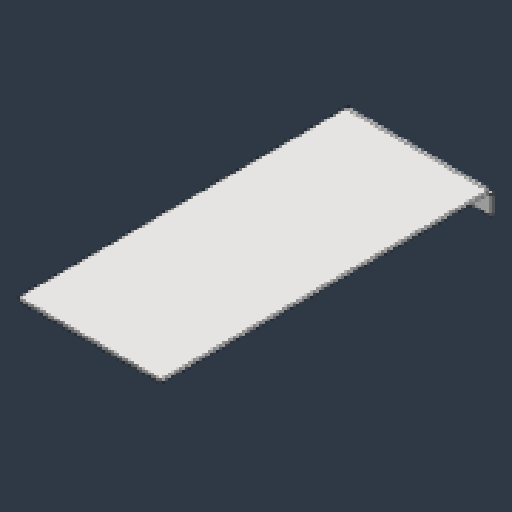
# Autodesk Inventor part: feeder_front_support
Saved by Autodesk Inventor 2024.3 (Build 283343000, 343)
## iProperties
Created: 2025-03-08
Part Number: feeder_front_support
Material: Polycarbonate, Smoke
Document SubType Name: Sheet Metal
Designer: marcu
Density: 1.2 g/cm^3
Sheet Metal Rule: Default
Appearance: Polycarbonate - Smoked
Author: marcu
Autodesk Inventor part; units mm, degrees
ref_plane "YZ Plane" through (0, 0, 0) normal (1, 0, 0) x (0, 1, 0)
ref_plane "XZ Plane" through (0, 0, 0) normal (0, 1, 0) x (-1, 0, 0)
ref_plane "XY Plane" through (0, 0, 0) normal (0, 0, 1) x (1, 0, 0)
sketch "Sketch1" plane through (0, 0, 0) normal (0, 0, 1) x (1, 0, 0)
  line L0 (76.2, -12.7) -> (-76.2, -12.7)
  line L1 (-76.2, -12.7) -> (-76.2, 12.7)
  line L2 (-76.2, 12.7) -> (76.2, 12.7)
  line L3 (76.2, 12.7) -> (76.2, -12.7)
  line L4 (76.2, -12.7) -> (-76.2, 12.7) construction
  line L5 (-76.2, -12.7) -> (76.2, 12.7) construction
  point P0 (0, 0)
  dimension "d0" = 152.4
  dimension "d1" = 25.4
  measures "d0" distance of L1.end L2.end
  measures "d1" distance of L0.end L1.end
extrude "Plate1" add sketch "Sketch1" along normal blind 3.048
sketch "Sketch2" plane through (-76.2, 9.652, 0) normal (0, 1, 0) x (-1, 0, 0)
  line L0 (-152.4, 0) -> (0, 0)
  line L1 (0, 0) -> (0, 336.55)
  line L2 (0, 336.55) -> (-152.4, 336.55)
  line L3 (-152.4, 336.55) -> (-152.4, 0)
  constraints: 6 end point, 1 horizontal, 1 perpendicular, 1 vertical
edge flange "Flange1" height 336.55 angle 90 thickness 3.048 bend radius 3.048 thickness toward (0, 1, 0) relief straight relief width 3.048 relief depth 1.524 edges at (0, 12.7, 3.048) wall of the first edge with corners at (76.2, 9.652, 0) (-76.2, 9.652, 0) (-76.2, 9.652, 336.55) (76.2, 9.652, 336.55)
bend "Bend1"
corner "Corner1"
sketch "Sketch3" plane through (0, 0, 3.048) normal (0, 0, 1) x (1, 0, 0)
  line L0 (76.2, 6.604) -> (-76.2, 6.604) construction
  line L1 (-76.2, -12.7) -> (-76.2, 6.604) construction
  line L2 (76.2, -12.7) -> (-76.2, -12.7) construction
  line L3 (76.2, 6.604) -> (76.2, -12.7) construction
  line L4 (0, 6.604) -> (0, -12.7) construction
  line L5 (0, 1.5875) -> (-6.35, 1.5875) construction
  point P0 (0, 0)
  point P1 (-31.75, 1.5875)
  point P2 (-57.15, 1.5875)
  point P3 (6.35, 1.5875)
  point P4 (31.75, 1.5875)
  point P5 (57.15, 1.5875)
  dimension "d13" = 6.35
  dimension "d16" = 25.4
  dimension "d28" = 14.2875
  constraints: 4 end point, 3 symmetric about line, 2 horizontal, 2 midpoint, 1 coincident, 2 other
  measures "d13" distance of L5.start L5.end
  measures "d16" distance of L5.end point (-31.75, 1.587)
  measures "d28" distance from line of L2 L5.start
hole "Hole1" at (-6.35, 1.5875, 3.048) at (6.35, 1.5875, 3.048) at (-31.75, 1.5875, 3.048) at (-57.15, 1.5875, 3.048) at (31.75, 1.5875, 3.048) at (57.15, 1.5875, 3.048) direction (0, 0, -1) diameter 5.1054 end through all clearance for "Flat Head Machine Screw (82)" size "#10" standard "Ansi Unified Screw Threads"
sketch "Sketch4" plane through (-76.2, 13.7425, 333.6858) normal (0, -0.3420201, 0.9396926) x (1, 0, 0)
  line L0 (152.4, 0) -> (0, 0)
  line L1 (0, 0) -> (0, -50.8)
  line L2 (0, -50.8) -> (152.4, -50.8)
  line L3 (152.4, -50.8) -> (152.4, 0)
  constraints: 6 end point, 1 horizontal, 1 perpendicular, 1 vertical
edge flange "Flange2" height 50.8 angle 110 thickness 3.048 bend radius 3.048 thickness toward (0, -0.3420201, 0.9396926) relief straight relief width 3.048 relief depth 1.524 edges at (0, 9.652, 336.55) wall of the first edge with corners at (76.2, 13.7425, 333.6858) (-76.2, 13.7425, 333.6858) (-76.2, -33.9939, 316.3112) (76.2, -33.9939, 316.3112)
bend "Bend2"
corner "Corner2"
equation "\"d26\" = Thickness"
equation "\"d2\" = Thickness"
equation "\"d3\" = BendReliefWidth"
equation "\"d4\" = BendReliefDepth"
equation "\"d5\" = MinimumRemnant"
equation "\"d6\" = TransitionRadius"
equation "\"d9\" = BendRadius"
equation "\"d10\" = CornerReliefSize"
equation "\"d11\" = GapSize"
equation "\"d12\" = JacobiRadiusSize"
equation "\"d29\" = BendReliefWidth"
equation "\"d30\" = BendReliefDepth"
equation "\"d31\" = MinimumRemnant"
equation "\"d32\" = TransitionRadius"
equation "\"d35\" = BendRadius"
equation "\"d36\" = CornerReliefSize"
equation "\"d37\" = GapSize"
equation "\"d38\" = JacobiRadiusSize"
equation "\"BendRadius\" = Thickness"
equation "\"BendReliefWidth\" = Thickness"
equation "\"BendReliefDepth\" = 0.5 * Thickness"
equation "\"CornerReliefSize\" = 4 * Thickness"
equation "\"MinimumRemnant\" = 2 * Thickness"
equation "\"TransitionRadius\" = BendRadius"
equation "\"JacobiRadiusSize\" = BendRadius"
equation "\"GapSize\" = Thickness"
equation "\"Thickness\" = 3.048"
body "Solid1"
